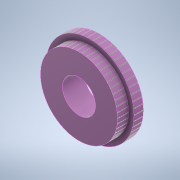
# Autodesk Inventor part: 1
Saved by Autodesk Inventor 2021 (Build 250183000, 183)
## iProperties
Created: 2022-06-28
Part Number: 1
Material: Пластик АБС
Document SubType Name: Modeling
Designer: termi
Density: 1.06 g/cm^3
Appearance: Гладкий - белый
Mass: 617.927 g
Surface Area: 648.484 cm^2
Volume: 582.95 cm^3
Author: termi
Autodesk Inventor part; units mm, degrees
ref_plane "YZ Plane" through (0, 0, 0) normal (1, 0, 0) x (0, 1, 0)
ref_plane "XZ Plane" through (0, 0, 0) normal (0, 1, 0) x (-1, 0, 0)
ref_plane "XY Plane" through (0, 0, 0) normal (0, 0, 1) x (1, 0, 0)
sketch "Эскиз1" plane through (0, 0, 0) normal (0, 1, 0) x (-1, 0, 0)
  line L0 (-30, 0) -> (-30, -40)
  line L1 (-30, 0) -> (-80, 0)
  line L2 (-80, 0) -> (-80, -40)
  line L3 (-80, -40) -> (-30, -40)
  line L4 (-30, -40) -> (-30, 0)
  line L5 (-80, 0) -> (-70, 0)
  line L6 (-70, 0) -> (-70, -20)
  line L7 (-70, -20) -> (-80, -20)
  line L8 (-80, -20) -> (-80, 0)
  line L9 (-80, -40) -> (-70, -40)
  line L10 (-70, -40) -> (-70, -37)
  line L11 (-70, -37) -> (-80, -37)
  line L12 (-80, -37) -> (-80, -40)
  line L13 (0, 21.2559) -> (0, -55.7525) construction
  point P0 (0, 0)
  dimension "d0" = 50
  dimension "d1" = 10
  dimension "d2" = 20
  dimension "d3" = 10
  dimension "d4" = 3
  dimension "d5" = 40
  constraints: 28 end point, 6 parallel, 3 horizontal, 3 perpendicular, 2 vertical, 1 point on line, 2 other
  measures "d0" distance of L3.end L2.end
  measures "d1" distance of L6.end L7.end
  measures "d2" distance of L5.end L6.end
  measures "d3" distance of L11.end L10.end
  measures "d4" distance of L10.end L9.end
  measures "d5" distance of L1.end L2.end
revolve "Вращение1" add sketch "Эскиз1" angle 360 about axis through (0, 0, 21.2559) along (0, 0, -1) contours L0 L3 L10 L11 L2 L7 L6 L1
sketch "Эскиз3" plane through (0, 0, 0) normal (0, 0, 1) x (1, 0, 0)
  line L0 (69.95, -0.5) -> (70.05, -0.5)
  line L1 (70.05, -0.5) -> (70.05, 0.5)
  line L2 (70.05, 0.5) -> (69.95, 0.5)
  line L3 (69.95, 0.5) -> (69.95, -0.5)
  circle A0 centre (0, 0) radius 70 projected
  line L4 (69.95, -0.5) -> (70.05, 0.5) construction
  line L5 (70.05, -0.5) -> (69.95, 0.5) construction
  line L6 (79.95, -0.5) -> (80.05, -0.5)
  line L7 (80.05, -0.5) -> (80.05, 0.5)
  line L8 (80.05, 0.5) -> (79.95, 0.5)
  line L9 (79.95, 0.5) -> (79.95, -0.5)
  circle A1 centre (0, 0) radius 80 projected
  line L10 (79.95, -0.5) -> (80.05, 0.5) construction
  line L11 (80.05, -0.5) -> (79.95, 0.5) construction
  point P0 (70, 0)
  point P1 (80, 0)
  dimension "d9" = 0.1
  dimension "d10" = 1
  dimension "d11" = 0.1
  dimension "d12" = 1
  constraints: 24 end point, 4 midpoint, 4 parallel, 2 horizontal, 2 horizontal alignment, 2 perpendicular, 2 other
  measures "d9" distance of L2.end L1.end
  measures "d10" distance of L1.end L0.end
  measures "d11" distance of L8.end L7.end
  measures "d12" distance of L7.end L6.end
extrude "Выдавливание1" add sketch "Эскиз3" against normal up to surface (20 mm away) separate body contours L3 L2 A0 L0 | A0 L2 L1 L0 picked at (69.9664, -0.1111)
sketch "Эскиз4" plane through (0, 0, -20) normal (0, 0, 1) x (1, 0, 0)
  line L0 (79.95, -0.5) -> (80.05, -0.5)
  line L1 (80.05, -0.5) -> (80.05, 0.5)
  line L2 (80.05, 0.5) -> (79.95, 0.5)
  line L3 (79.95, 0.5) -> (79.95, -0.5)
  circle A0 centre (0, 0) radius 80 projected
  line L4 (79.95, -0.5) -> (80.05, 0.5) construction
  line L5 (80.05, -0.5) -> (79.95, 0.5) construction
  point P0 (80, 0)
  dimension "d15" = 0.1
  dimension "d16" = 1
  constraints: 12 end point, 2 midpoint, 2 parallel, 1 horizontal, 1 horizontal alignment, 1 perpendicular, 1 other
  measures "d15" distance of L2.end L1.end
  measures "d16" distance of L1.end L0.end
extrude "Выдавливание2" add sketch "Эскиз4" against normal up to surface (17 mm away) contours L3 L2 A0 L0 | A0 L2 L1 L0 picked at (79.9664, -0.1111) bodies 2
pattern_circular "Круговой массив1" count 50 over 360 about axis through (0, 0, -10) along (0, 0, 1) of "Выдавливание1", "Выдавливание2" bodies 2
